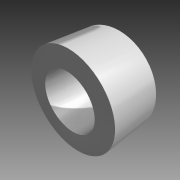
# Autodesk Inventor part: abstandshalter
Saved by Autodesk Inventor 2013 (Build 170138000, 138)
## iProperties
Created: 2012-10-19
Part Number: abstandshalter
Material: Aluminium
Document SubType Name: Modeling
Designer: fivef
Density: 2.71 g/cm^3
Mass: 0.681097 g
Surface Area: 3.51858 cm^2
Volume: 0.251327 cm^3
Author: fivef
Autodesk Inventor part; units mm, degrees
ref_plane "YZ Plane" through (0, 0, 0) normal (1, 0, 0) x (0, 1, 0)
ref_plane "XZ Plane" through (0, 0, 0) normal (0, 1, 0) x (-1, 0, 0)
ref_plane "XY Plane" through (0, 0, 0) normal (0, 0, 1) x (1, 0, 0)
sketch "Skizze1" plane through (0, 0, 0) normal (0, 1, 0) x (-1, 0, 0)
  circle A0 centre (0, 0) radius 5
  circle A1 centre (0, 0) radius 3
  dimension "d0" = 2
  dimension "d2" = 10
  dimension "d20" = 6
  constraints: 2 centre point, 2 coincident
  measures "d0" radial gap between concentric circles of A0 A1
  measures "d2" diameter of A0
  measures "d20" diameter of A1
extrude "Extrusion1" add sketch "Skizze1" along normal mid plane 5
